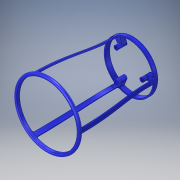
# Autodesk Inventor part: Form
Saved by Autodesk Inventor 2019.1 (Build 231200000, 200)
## iProperties
Created: 2018-07-22
Part Number: Form
Material: Generisch
Document SubType Name: Modeling
Designer: JochenAlt
Density: 1 g/cm^3
Appearance: Textur - grau
Author: JochenAlt
Autodesk Inventor part; units mm, degrees
ref_plane "YZ Plane" through (0, 0, 0) normal (1, 0, 0) x (0, 1, 0)
ref_plane "XZ Plane" through (0, 0, 0) normal (0, 1, 0) x (-1, 0, 0)
sketch "Skizze3" plane through (0, 0, 0) normal (0, 0, 1) x (1, 0, 0)
  line L0 (0, 276.9941) -> (0, -256.1657) construction
  line L1 (-139.25, 0) -> (205.5, 0) construction
  circle A0 centre (0, 0) radius 90 construction
  circle A1 centre (0, -90) radius 90 construction
  line L2 (153.75, 101.6438) -> (156.25, 101.6438) construction
  line L3 (63.6396, 63.6396) -> (107.1267, 107.1267) construction
  line L4 (63.6396, -26.3604) -> (107.1267, 17.1267) construction
  circle A2 centre (107.1267, 17.1267) radius 8.5 construction
  circle A3 centre (107.1267, 107.1267) radius 8.5 construction
  line L5 (105, -90) -> (90, -90) construction
  line L6 (115.2082, 109.7607) -> (119.9621, 111.3102) construction
  arc A4 (109.3117, 123.4538) -> (109.3117, 144.667) centre (98.7051, 134.0604) ccw construction
  line L7 (109.3117, 123.4538) -> (65.9557, 80.0979) construction
  spline S0 degree 4 poles (105, -80) (105, 8.897) (92.8492, 72.1883) (84, 108.2247) (84, 170) knots 1.030471 1.030471 1.030471 1.030471 1.030471 1.953705 1.953705 1.953705 1.953705 1.953705
  line L8 (80, 200) -> (-80, 200) construction
  line L9 (-80, 110) -> (80, 110) construction
  line L10 (80, 200) -> (80, 200)
  line L11 (84, 196) -> (84, 185)
  arc A5 (84, 196) -> (80, 200) centre (80, 196) ccw
  line L12 (0, -80) -> (0, 185)
  line L13 (0, -80) -> (101, -80)
  line L14 (105, -80) -> (105, 8.897) construction
  line L15 (101, -90) -> (101, -80)
  arc A6 (101, -90) -> (105, -80) centre (105, -85.8) ccw
  line L16 (101, -80) -> (105, -80)
  line L17 (105, 8.897) -> (92.8492, 72.1883) construction
  line L18 (92.8492, 72.1883) -> (84, 108.2247) construction
  line L19 (84, 108.2247) -> (84, 170) construction
  line L20 (80, 185) -> (0, 185)
  line L21 (80, 200) -> (80, 185)
  line L22 (80, 185) -> (84, 185)
  line L23 (84, 170) -> (84, 185)
  point P0 (84, 200)
  dimension "d13" = 180
  dimension "d108" = 17
  dimension "d14" = 90
  dimension "d106" = 61.5
  dimension "d107" = 45
  dimension "d110" = 15
  dimension "d112" = 5
  dimension "d119" = 10
  dimension "d120" = 15
  dimension "d204" = 200
  dimension "d206" = 200
  dimension "d207" = 4
  dimension "d209" = 4
  dimension "d210" = 160
  dimension "d220" = 4
  dimension "d224" = 10
  dimension "d227" = 15
  dimension "d230" = 4
  constraints: 36 end point, 10 point on circle, 10 point on line, 7 horizontal, 6 perpendicular, 4 centre point, 4 parallel, 3 coincident, 3 tangent, 2 symmetric about line, 1 collinear, 1 line through centre, 1 vertical, 18 other
  measures "d14" distance of A1.centre point (0, 0)
  measures "d106" distance of L3.start L3.end
  measures "d107" angle of L0 L3
  measures "d110" distance of L5.start L5.end
  measures "d112" distance of L6.start L6.end
  measures "d119" distance from line of L7.start L3
  measures "d120" radius of A4
  measures "d204" distance from line of L8 point (0, 0)
  measures "d206" distance from line of A1.centre L9
  measures "d207" distance of L8.start point (84, 200)
  measures "d209" radius of A5
  measures "d210" distance of L8.start L8.end
  measures "d220" distance of L15.start L5.start
  measures "d224" distance of L15.start L13.end
  measures "d227" vertical distance of L11.end L8.start
  measures "d230" distance from line of L14 L13.end
revolve "Umdrehung1" add sketch "Skizze3" angle 360 about axis through (0, 0, 0) along (0, -1, 0) contours L16 L13 L12 L20 L22 L23 S0
shell "Wandung1" thickness 4 removed faces 4 at (-102.1693, -80, 0) at (31.1641, -80, 16.0077) at (23.7602, 185, -12.1064) at (-80.9229, 185, -6.315)
sketch "Skizze11" plane through (0, 0, 0) normal (0, 1, 0) x (-1, 0, 0)
  line L0 (0, -211.1576) -> (0, 211.1576) construction
  line L1 (-196, 0) -> (196, 0) construction
  line L2 (26.6571, -39.5208) -> (78.287, -116.0653)
  line L3 (26.6571, 39.5208) -> (78.287, 116.0653)
  line L4 (20.8974, 42.8461) -> (61.372, 125.8312)
  line L5 (-47.5546, 3.3253) -> (-139.659, 9.7659)
  line L6 (-47.5546, -3.3253) -> (-139.659, -9.7659)
  line L7 (20.8974, -42.8461) -> (61.372, -125.8312)
  arc A0 (-139.659, -9.7659) -> (61.372, -125.8312) centre (0, 0) ccw
  arc A1 (78.287, -116.0653) -> (78.287, 116.0653) centre (0, 0) ccw
  arc A2 (61.372, 125.8312) -> (-139.659, 9.7659) centre (0, 0) ccw
  arc A3 (26.6571, -39.5208) -> (26.6571, 39.5208) centre (0, 0) ccw
  arc A4 (20.8974, 42.8461) -> (-47.5546, 3.3253) centre (0, 0) ccw
  arc A5 (-47.5546, -3.3253) -> (20.8974, -42.8461) centre (0, 0) ccw
  line L8 (0, 0) -> (62.9066, -108.9574) construction
  dimension "d217" = 140
  dimension "d241" = 8
  dimension "d242" = 8
  dimension "d243" = 8
  dimension "d246" = 120
  constraints: 14 end point, 12 point on circle, 6 centre point, 6 point on line, 4 concentric, 2 coincident, 3 other
  measures "d217" radius of A1
  measures "d241" angle of L3 L4
  measures "d242" angle of L2 L7
  measures "d243" angle of L6 L5
  measures "d246" angle of L1 L8
extrude "Extrusion23" add sketch "Skizze11" against normal up to surface (265 mm away) from surface at 185 separate body
fillet "Rundung6" radius 5 12 edges at (-41.1347, 185, -84.3386) (93.6068, 185, -6.5456) (-52.4721, 185, -77.793) (-52.4721, 185, 77.793) (-41.1347, 185, 84.3386) (93.6068, 185, 6.5456) (93.6068, -80, 6.5456) (-52.4721, -80, -77.793) (93.6068, -80, -6.5456) (-41.1347, -80, 84.3386) (-52.4721, -80, 77.793) (-41.1347, -80, -84.3386)
revolve "Umdrehung2" add sketch "Skizze3" angle 360 about axis through (0, 0, 0) along (0, -1, 0) bodies 1 contours A6 L15 L16
combine bodies "Kombinieren5" operation type subtract main body 1 bodies to subtract 2
revolve "Umdrehung3" add sketch "Skizze3" angle 360 about axis through (0, 0, 0) along (0, -1, 0) bodies 1 contours A6 L15 L16 | L22 L21 A5 L11
ref_plane "Arbeitsebene3" through (80, 200, 0) normal (0, 1, 0) x (-1, 0, 0)
sketch "Skizze7" plane through (0, 200, 0) normal (0, 1, 0) x (-1, 0, 0)
  arc A0 (-56.5733, -7.0393) -> (-56.5733, 7.0393) centre (-57.5, 0) ccw
  circle A1 centre (-57.5, 0) radius 4.1
  line L0 (0, -112) -> (0, 112) construction
  line L1 (-37.4, -64.7787) -> (-37.4, -64.7787)
  arc A2 (-63.6619, -11.7905) -> (-63.6619, -11.7905) centre (0, 0) ccw
  arc A3 (-59, -5.9127) -> (-56, -5.9127) centre (-57.5, 0) ccw
  arc A4 (-56, 5.9127) -> (-59, 5.9127) centre (-57.5, 0) ccw
  arc A5 (-56, -4.8744) -> (-56, 4.8744) centre (-57.5, 0) ccw
  arc A6 (-59, 4.8744) -> (-59, -4.8744) centre (-57.5, 0) ccw
  line L2 (-56, -5.9127) -> (-56, -4.8744)
  line L3 (-56, 4.8744) -> (-56, 5.9127)
  line L4 (-59, -5.9127) -> (-59, -4.8744)
  line L5 (-59, 4.8744) -> (-59, 5.9127)
  line L6 (-57.5, -6.1) -> (-57.5, 6.1) construction
  arc A7 (-79.3675, 10.0402) -> (-79.3675, -10.0402) centre (0, 0) ccw
  line L7 (-112, 0) -> (112, 0) construction
  circle A8 centre (0, 0) radius 80 projected
  line L8 (-79.3675, 10.0402) -> (-56.5733, 7.0393)
  line L9 (-56.5733, -7.0393) -> (-79.3675, -10.0402)
  circle A9 centre (0, 0) radius 80 projected
  arc A10 (-56.5733, 7.0393) -> (-56.5733, -7.0393) centre (-57.5, 0) ccw
  dimension "d142" = 57.5
  dimension "d196" = 10.2
  dimension "d197" = 1
  dimension "d199" = 3
  dimension "d200" = 12.2
  dimension "d201" = 2
  dimension "d229" = 15
  constraints: 18 point on circle, 16 end point, 9 centre point, 5 coincident, 5 vertical, 3 point on line, 2 collinear, 2 concentric, 2 midpoint, 2 tangent, 4 other
  measures "d142" distance of A0.centre point (0, 0)
  measures "d196" diameter of A5
  measures "d197" radial gap between concentric circles of A1 A5
  measures "d199" distance between parallel lines of L4 L2
  measures "d200" diameter of A3
  measures "d201" radial gap between concentric circles of A0 A5
  measures "d229" angle of L9 L8
extrude "Extrusion5" add sketch "Skizze7" against normal blind 30 separate body contours A10 A0 | L9 A2 L8 A10 | L9 A7 L8 A2
extrude "Extrusion8" add sketch "Skizze7" along normal blind 2 from surface at -30 contours L4 A6 L5 A4 L3 A5 L2 A3 bodies 3
extrude "Extrusion25" cut sketch "Skizze7" along normal blind 15 from surface at -30 contours L9 A2 L8 A10 | L9 A7 L8 A2 bodies 1 3
pattern_circular "Runde Anordnung2" count 3 over 360 about axis through (0, -10, 0) along (0, 1, 0) bodies 3
combine bodies "Kombinieren3" operation type add bodies to combine 1 3
equation "\"d14\" = 0.5 * d13"
